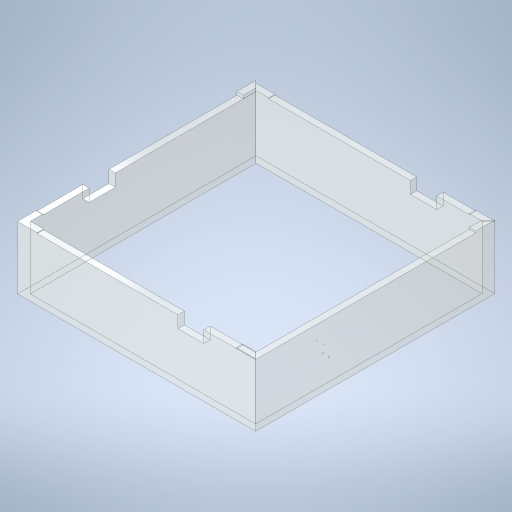
# Autodesk Inventor part: Exterior_Walls
Saved by Autodesk Inventor 2024 (Build 280153000, 153)
## iProperties
Created: 2023-05-16
Part Number: Exterior_Walls
Material: Concrete
Document SubType Name: Modeling
Designer: Tom
Density: 2.40731 g/cm^3
Appearance: Clear
Mass: 3.19414e+07 g
Surface Area: 1.46557e+06 cm^2
Volume: 1.32685e+07 cm^3
Author: Tom
Autodesk Inventor part; units mm, degrees
ref_plane "YZ Plane" through (0, 0, 0) normal (1, 0, 0) x (0, 1, 0)
ref_plane "XZ Plane" through (0, 0, 0) normal (0, 1, 0) x (-1, 0, 0)
ref_plane "XY Plane" through (0, 0, 0) normal (0, 0, 1) x (1, 0, 0)
sketch "Sketch1" plane through (0, 0, 0) normal (0, 1, 0) x (-1, 0, 0)
  line L0 (0, 0) -> (12.7, 7213.5888)
  line L1 (12.7, 7213.5888) -> (7200.9, 7213.5888)
  line L2 (7200.9, 7213.5888) -> (7213.6, 0)
  line L3 (7213.6, 0) -> (0, 0)
  line L4 (7403.7426, 7416.7888) -> (-190.1426, 7416.7888)
  line L5 (-190.1426, 7416.7888) -> (-203.5581, -203.2)
  line L6 (-203.5581, -203.2) -> (7417.1581, -203.2)
  line L7 (7417.1581, -203.2) -> (7403.7426, 7416.7888)
  dimension "d1" = 7188.2
  dimension "d3" = 12.7
  dimension "d4" = 7213.6
  dimension "d5" = 7213.6
  dimension "d6" = 203.2
  dimension "d8" = 7213.6
  constraints: 16 end point, 1 horizontal, 3 other
  measures "d1" distance of L0.end L1.end
  measures "d3" horizontal distance of L0.start L0.end
  measures "d4" distance of L1.end L2.end
  measures "d5" distance of L2.end L0.start
  measures "d6" distance between parallel lines of L4 L1
  measures "d8" distance of L0.start L0.end
extrude "Extrusion1" add sketch "Sketch1" along normal blind 1981.2
sketch "Sketch3" plane through (-12.7, 0, 7213.5888) normal (0, 0, -1) x (-1, 0, 0)
  line L0 (7391.0426, 1981.2) -> (-202.8426, 1981.2) projected
  line L1 (2273.3, 2006.6) -> (2273.3, 1600.2)
  line L2 (2273.3, 1600.2) -> (1447.8, 1600.2)
  line L3 (1447.8, 1600.2) -> (1447.8, 2006.6)
  line L4 (0, 0) -> (0, 1981.2) projected
  line L5 (0, 0) -> (7188.2, 0) projected
  line L6 (1447.8, 2006.6) -> (2273.3, 2006.6)
  point P0 (-12.7, 0)
  dimension "d20" = 1447.8
  dimension "d102" = 825.5
  dimension "d103" = 406.4
  dimension "d104" = 25.4
  constraints: 8 end point, 1 horizontal, 1 parallel, 1 perpendicular
  measures "d20" distance between parallel lines of L4 L3
  measures "d102" distance of L3.end L1.start
  measures "d103" distance of L2.end L3.end
  measures "d104" distance between parallel lines of L0 L6
extrude "Extrusion2" cut sketch "Sketch3" against normal up to surface (203.2 mm away)
sketch "Sketch4" plane through (-12.7, 0, 7213.5888) normal (-0.9999985, 0, -0.0017606) x (-0.0017606, 0, 0.9999985)
  line L0 (-7213.6, 0) -> (0, 0) projected
  line L1 (-7213.6, 0) -> (-7213.6, 1981.2) projected
  point P0 (-1955.8, 1330.325)
  dimension "d27" = 1330.325
  dimension "d28" = 5257.8
  measures "d27" distance from line of L0 point (-1955.8, 1330.325)
  measures "d28" distance from line of L1 point (-1955.8, 1330.325)
hole "Hole1" at (-9.2567, 1330.325, 5257.7919) direction (0.9999985, 0, 0.0017606) diameter 19.05 end through all
sketch "Sketch5" plane through (-12.7, 0, 7213.5888) normal (-0.9999985, 0, -0.0017606) x (-0.0017606, 0, 0.9999985)
  line L0 (-7213.6, 0) -> (0, 0) projected
  line L1 (-7213.6, 0) -> (-7213.6, 1981.2) projected
  point P0 (-2133.6, 889)
  dimension "d36" = 889
  dimension "d37" = 5080
  measures "d36" distance from line of L0 point (-2133.6, 889)
  measures "d37" distance from line of L1 point (-2133.6, 889)
hole "Hole2" at (-8.9437, 889, 5079.9921) direction (0.9999985, 0, 0.0017606) diameter 50.8 end through all
sketch "Sketch6" plane through (-7213.6, 0, 0) normal (0, 0, 1) x (1, 0, 0)
  line L0 (7417.1581, 1981.2) -> (-203.5581, 1981.2) projected
  line L1 (7213.6, 0) -> (7213.6, 1981.2) projected
  line L2 (0, 0) -> (7213.6, 0) projected
  line L3 (5765.8, 1600.2) -> (4927.6, 1600.2)
  line L4 (4927.6, 1600.2) -> (4927.6, 2006.6)
  line L5 (4927.6, 2006.6) -> (5765.8, 2006.6)
  line L6 (5765.8, 2006.6) -> (5765.8, 1600.2)
  dimension "d105" = 406.4
  dimension "d106" = 1447.8
  dimension "d107" = 838.2
  dimension "d108" = 25.4
  constraints: 8 end point, 2 parallel, 1 horizontal, 1 perpendicular
  measures "d105" distance of L3.end L4.end
  measures "d106" distance from line of L1.end L6
  measures "d107" distance of L3.start L3.end
  measures "d108" distance between parallel lines of L0 L5
extrude "Extrusion3" cut sketch "Sketch6" against normal up to surface (203.2 mm away)
sketch "Sketch8" plane through (-7200.9, 0, 7213.5888) normal (0.9999985, 0, -0.0017606) x (-0.0017606, 0, -0.9999985)
  line L0 (2717.8, 2070.1) -> (1879.6, 2070.1)
  line L1 (1879.6, 2070.1) -> (1879.6, 1587.5)
  line L2 (1879.6, 1587.5) -> (2717.8, 1587.5)
  line L3 (2717.8, 1587.5) -> (2717.8, 2070.1)
  line L4 (0, 0) -> (0, 1981.2) projected
  line L5 (0, 0) -> (7213.6, 0) projected
  point P0 (7200.9, 0)
  point P1 (4368.8, 0)
  dimension "d56" = 2717.8
  dimension "d118" = 1587.5
  dimension "d119" = 482.6
  dimension "d120" = 838.2
  constraints: 8 end point, 2 parallel, 1 horizontal, 1 perpendicular
  measures "d56" distance between parallel lines of L4 L3
  measures "d118" distance between parallel lines of L5 L2
  measures "d119" distance of L0.end L1.end
  measures "d120" distance of L0.start L0.end
extrude "Extrusion5" cut sketch "Sketch8" against normal up to surface (203.2 mm away)
sketch "Sketch13" plane through (0, 1981.2, 0) normal (0, 1, 0) x (1, 0, 0)
  line L0 (0, 0) -> (-12.7, -7213.5888) projected
  line L1 (190.1426, -7416.7888) -> (203.5581, 203.2) projected
  line L2 (0, 0) -> (203.5581, 203.2)
  line L3 (203.5581, 203.2) -> (202.4848, -406.4)
  line L4 (-0.7149, -406.0423) -> (0, 0)
  line L5 (-0.7149, -406.0423) -> (202.4848, -406.4)
  dimension "d84" = 609.6
  constraints: 8 end point, 2 perpendicular, 1 parallel, 1 point on line
  measures "d84" distance of L1.end L3.end
extrude "Extrusion9" add sketch "Sketch13" along normal blind 50.8
sketch "Sketch14" plane through (0, 1981.2, 0) normal (0, 1, 0) x (1, 0, 0)
  line L0 (190.1426, -7416.7888) -> (203.5581, 203.2) projected
  line L1 (0, 0) -> (-12.7, -7213.5888) projected
  line L2 (190.1426, -7416.7888) -> (-12.7, -7213.5888)
  line L3 (-12.7, -7213.5888) -> (-419.1003, -7212.8733)
  line L4 (-419.1003, -7212.8733) -> (-419.4574, -7415.7156)
  line L5 (-419.4574, -7415.7156) -> (190.1426, -7416.7888)
  line L6 (-7403.7426, -7416.7888) -> (-2286, -7416.7888) projected
  line L7 (-12.7, -7213.5888) -> (-7200.9, -7213.5888) projected
  line L8 (-7403.7426, -7416.7888) -> (-7200.9, -7213.5888)
  line L9 (-7403.7426, -7416.7888) -> (-6776.6052, -7416.7888)
  line L10 (-7200.9, -7213.5888) -> (-6776.6052, -7213.5888)
  line L11 (-6776.6052, -7213.5888) -> (-6776.6052, -7416.7888)
  point P0 (202.4848, -406.4)
  point P1 (-0.7149, -406.0423)
  dimension "d87" = 609.6
  dimension "d91" = 627.1374
  constraints: 16 end point, 4 perpendicular, 2 collinear
  measures "d87" distance of L4.end L0.start
  measures "d91" distance of L6.start L9.end
extrude "Extrusion10" add sketch "Sketch14" along normal blind 25.4
sketch "Sketch15" plane through (0, 1981.2, 0) normal (0, 1, 0) x (1, 0, 0)
  line L0 (-7200.9, -7213.5888) -> (-7403.7426, -7416.7888) projected
  line L1 (-7403.7426, -7416.7888) -> (-7200.9, -7213.5888)
  line L2 (-7200.9, -7213.5888) -> (-7201.6161, -6806.8311)
  line L3 (-7200.9, -7213.5888) -> (-7213.6, 0) projected
  line L4 (-7201.6161, -6806.8311) -> (-7404.8158, -6807.1888)
  line L5 (-7417.1581, 203.2) -> (-7403.7426, -7416.7888) projected
  line L6 (-7404.8158, -6807.1888) -> (-7403.7426, -7416.7888)
  point P0 (0, 0)
  point P1 (-7208.5915, -2844.7956)
  point P2 (-7411.7912, -2845.1533)
  dimension "d92" = 609.6
  constraints: 8 end point, 3 point on line, 2 perpendicular, 1 collinear
  measures "d92" distance of L4.end L6.end
extrude "Extrusion11" add sketch "Sketch15" along normal blind 25.4
sketch "Sketch16" plane through (0, 1981.2, 0) normal (0, 1, 0) x (1, 0, 0)
  line L0 (203.5581, 203.2) -> (-7417.1581, 203.2) projected
  line L1 (-7213.6, 0) -> (0, 0) projected
  line L2 (-7417.1581, 203.2) -> (-7213.6, 0)
  line L3 (-7213.6, 0) -> (-7213.6, -406.4)
  line L4 (-7213.6, -406.4) -> (-7416.0848, -406.4)
  line L5 (-7417.1581, 203.2) -> (-7403.7426, -7416.7888) projected
  line L6 (-7417.1581, 203.2) -> (-7416.0848, -406.4)
  point P0 (-7415.011, -1016.3562)
  dimension "d95" = 609.6
  constraints: 8 end point, 2 perpendicular, 1 collinear, 1 point on line
  measures "d95" distance of L0.end L4.end
extrude "Extrusion12" add sketch "Sketch16" along normal blind 101.6
sketch "Sketch17" plane through (0, 1981.2, 0) normal (0, 1, 0) x (1, 0, 0)
  line L0 (-7417.1581, 203.2) -> (-7403.7426, -7416.7888) projected
  line L1 (-7417.1581, 203.2) -> (-7213.6, 0) projected
  line L2 (-7417.1581, 203.2) -> (-7213.6, 0)
  line L3 (-7213.6, 0) -> (-6807.5581, 0)
  line L4 (-7213.6, 0) -> (0, 0) projected
  line L5 (-6807.5581, 0) -> (-6807.5581, 203.2)
  line L6 (203.5581, 203.2) -> (-7417.1581, 203.2) projected
  line L7 (-6807.5581, 203.2) -> (-7417.1581, 203.2)
  line L8 (0, 0) -> (203.5581, 203.2) projected
  line L9 (203.5581, 203.2) -> (0, 0)
  line L10 (0, 0) -> (-406.0419, 0)
  line L11 (-406.0419, 0) -> (-406.0419, 203.2)
  line L12 (-406.0419, 203.2) -> (203.5581, 203.2)
  point P0 (-7415.011, -1016.3562)
  dimension "d98" = 609.6
  dimension "d99" = 609.6
  constraints: 16 end point, 5 point on line, 3 collinear, 3 perpendicular
  measures "d98" distance of L5.end L7.end
  measures "d99" distance of L11.end L6.start
extrude "Extrusion13" add sketch "Sketch17" along normal blind 25.4 contours L6 L5 L3 L1 | L6 L8 L4 L11
ref_plane "Work Plane2" through (-7200.9, 0, 7213.5888) normal (-1, 0, 0) x (0, 1, 0)
body "Solid1"
